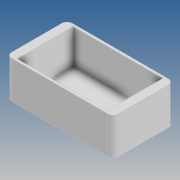
# Autodesk Inventor part: project_box
Saved by Autodesk Inventor 2020 (Build 240168000, 168)
## iProperties
Created: 2021-04-15
Part Number: project_box
Material: Generic
Document SubType Name: Modeling
Designer: stephen
Density: 1 g/cm^3
Appearance: Default
Author: stephen
Autodesk Inventor part; units mm, degrees
ref_plane "YZ Plane" through (0, 0, 0) normal (1, 0, 0) x (0, 1, 0)
ref_plane "XZ Plane" through (0, 0, 0) normal (0, 1, 0) x (-1, 0, 0)
ref_plane "XY Plane" through (0, 0, 0) normal (0, 0, 1) x (1, 0, 0)
sketch "Sketch1" plane through (0, 0, 0) normal (0, 1, 0) x (-1, 0, 0)
  line L0 (-78.994, -44.958) -> (78.994, -44.958)
  line L1 (78.994, -44.958) -> (78.994, 44.958)
  line L2 (78.994, 44.958) -> (-78.994, 44.958)
  line L3 (-78.994, 44.958) -> (-78.994, -44.958)
  line L4 (-78.994, -44.958) -> (78.994, 44.958) construction
  line L5 (78.994, -44.958) -> (-78.994, 44.958) construction
  point P0 (0, 0)
  dimension "d0" = 89.916
  dimension "d1" = 157.988
  constraints: 12 end point, 2 midpoint, 2 parallel, 1 horizontal, 1 perpendicular
  measures "d0" distance of L2.end L0.start
  measures "d1" distance of L1.end L2.end
extrude "Extrusion1" add sketch "Sketch1" along normal blind 55.118
fillet "Fillet1" radius 7.62 4 edges at (78.994, 27.559, 44.958) (78.994, 27.559, -44.958) (-78.994, 27.559, 44.958) (-78.994, 27.559, -44.958)
shell "Shell1" thickness 3.556 removed faces 1 at (23.7913, 55.118, -14.986)
sketch "Sketch2" plane through (-71.374, 3.556, 41.402) normal (0, 1, 0) x (1, 0, 0)
  line L0 (0, 0) -> (142.748, 0) projected
  line L1 (137.922, 0) -> (137.922, 82.804)
  line L2 (0, 82.804) -> (142.748, 82.804) projected
  line L3 (4.826, 82.804) -> (4.826, 0)
  line L4 (142.748, 0) -> (0, 0) projected
  line L5 (-4.064, 4.064) -> (-4.064, 78.74) projected
  line L6 (146.812, 78.74) -> (146.812, 4.064) projected
  arc A0 (0, 82.804) -> (-4.064, 78.74) centre (0, 78.74) ccw projected
  line L7 (-4.064, 78.74) -> (-4.064, 4.064) projected
  arc A1 (-4.064, 4.064) -> (0, 0) centre (0, 4.064) ccw projected
  line L8 (0, 0) -> (142.748, 0) projected
  arc A2 (142.748, 0) -> (146.812, 4.064) centre (142.748, 4.064) ccw projected
  line L9 (146.812, 4.064) -> (146.812, 78.74) projected
  arc A3 (146.812, 78.74) -> (142.748, 82.804) centre (142.748, 78.74) ccw projected
  line L10 (142.748, 82.804) -> (0, 82.804) projected
  point P0 (71.374, 41.402)
  point P1 (4.826, 0)
  point P2 (0, 82.804)
  point P3 (-4.064, 78.74)
  dimension "d6" = 133.096
  dimension "d7" = 8.89
  dimension "d8" = 8.89
  constraints: 4 end point, 4 point on line, 2 vertical
  measures "d6" distance between parallel lines of L1 L3
  measures "d7" distance between parallel lines of L3 L5
  measures "d8" distance between parallel lines of L1 L6
extrude "Extrusion2" add sketch "Sketch2" along normal up to surface (51.562 mm away) contours A1 L5 A0 L2 L3 L0 | L1 L2 A3 L6 A2 L0
equation "\"d7\" = d8"
body "Solid1"
